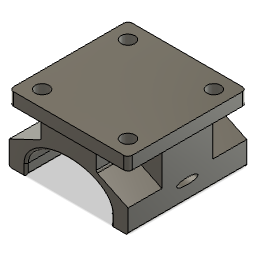
IMU_Thumb_Mount_03 v2 (Autodesk Fusion 360 design; units mm, degrees)
Autodesk Fusion 360 part; units mm, degrees
sketch "Sketch1" plane through (0, 0, 0) normal (0, 1, 0) x (1, 0, 0)
  line L0 (14, 14) -> (-14, 14)
  line L1 (-14, 14) -> (-14, -14)
  line L2 (-14, -14) -> (14, -14)
  line L3 (14, -14) -> (14, 14)
  line L4 (14, 14) -> (-14, -14) construction
  line L5 (-14, 14) -> (14, -14) construction
  line L6 (13, 13) -> (-13, 13) construction
  line L7 (-13, 13) -> (-13, -13) construction
  line L8 (-13, -13) -> (13, -13) construction
  line L9 (13, -13) -> (13, 13) construction
  line L10 (13, 13) -> (-13, -13) construction
  line L11 (-13, 13) -> (13, -13) construction
  line L12 (-10.125, 14) -> (-10.125, -14) construction
  line L13 (10.125, -14) -> (10.125, 14) construction
  line L14 (14, 10.125) -> (-14, 10.125) construction
  line L15 (-14, -10.125) -> (14, -10.125) construction
  circle A0 centre (10.125, 10.125) radius 1.625
  circle A1 centre (-10.125, 10.125) radius 1.625
  circle A2 centre (-10.125, -10.125) radius 1.625
  circle A3 centre (10.125, -10.125) radius 1.625
  dimension "d1" = 28
  dimension "d2" = 28
  dimension "d3" = 26
  dimension "d4" = 26
  dimension "d5" = 3.875
  dimension "d6" = 3.875
  dimension "d7" = 3.875
  dimension "d8" = 3.875
  dimension "d9" = 3.25
  dimension "d10" = 3.25
  dimension "d11" = 3.25
  dimension "d12" = 3.25
  constraint horizontal L0
  constraint perpendicular L0 L1
  constraint parallel L0 L2
  constraint parallel L1 L3
  constraint coincident L4 origin
  constraint coincident L5 origin
  constraint horizontal L6
  constraint perpendicular L6 L7
  constraint parallel L6 L8
  constraint parallel L7 L9
  constraint coincident L10 origin
  constraint coincident L11 origin
  constraint coincident L0 L12.start
  constraint coincident L2 L12.end
  constraint perpendicular L2 L12
  constraint coincident L2 L13.start
  constraint coincident L0 L13.end
  constraint perpendicular L0 L13
  constraint coincident L3 L14.start
  constraint perpendicular L3 L14
  constraint coincident L1 L14.end
  constraint coincident L1 L15.start
  constraint perpendicular L1 L15
  constraint coincident L3 L15.end
  constraint coincident L14 A0.centre
  constraint coincident L4 A0.centre
  constraint coincident L11 A1.centre
  constraint coincident L14 A1.centre
  constraint coincident L15 A2.centre
  constraint coincident L4 A2.centre
  constraint coincident L13 A3.centre
  constraint coincident L11 A3.centre
  measures "d1" distance of L1.end L2.end
  measures "d2" distance of L0.end L1.end
  measures "d3" distance of L7.end L8.end
  measures "d4" distance of L6.end L7.end
  measures "d5" distance of L3 L13
  measures "d6" distance of L1 L12
  measures "d7" distance of L2 L15
  measures "d8" distance of L0 L14
  measures "d9" diameter of A0
  measures "d10" diameter of A1
  measures "d11" diameter of A2
  measures "d12" diameter of A3
extrude "Extrude1" add sketch "Sketch1" along normal blind 3 makes body 1
sketch "Sketch2" plane through (0, 0, 0) normal (0, 0, 1) x (1, 0, 0)
  line L0 (0, 0) -> (0, -13) construction
  line L1 (0, 0) -> (0, -4.3333) construction
  line L2 (0, -13) -> (8.6667, -13)
  line L3 (0, -13) -> (-8.6667, -13)
  line L4 (-14, 0) -> (14, 0)
  line L5 (-8.5, 0) -> (-11.75, 0)
  line L6 (11.75, 0) -> (8.5, 0)
  line L7 (11.75, 0) -> (8.5, 0)
  line L8 (-8.5, 0) -> (-11.75, 0)
  line L9 (8.5, 0) -> (11.75, 0) construction
  line L10 (-8.5, 0) -> (-11.75, 0) construction
  line L11 (-8.5, 0) -> (-6.5, 0) construction
  line L12 (-11.75, 0) -> (-13.75, 0) construction
  line L13 (8.5, 0) -> (6.5, 0) construction
  line L14 (11.75, 0) -> (13.75, 0) construction
  line L15 (-6.5, 0) -> (-6.5, -7.1713)
  line L16 (6.5, 0) -> (6.5, -7.2675)
  line L17 (-6.5, -7.1713) -> (-13.755, -7.1713)
  line L18 (6.5, -7.2675) -> (13.8418, -7.2675)
  line L19 (0, -4.3333) -> (0, -10.3333) construction
  ellipse E0 centre (0, -10.3333) end of major axis (0, -4.3333) minor radius 10
  line L20 (0, -16.3333) -> (0, -4.3333) construction
  line L21 (10, -10.3333) -> (-10, -10.3333) construction
  line L22 (-10, -10.3333) -> (-14.8306, -10.3333) construction
  line L23 (10, -10.3333) -> (15, -10.3333) construction
  line L24 (14, 0) -> (14, -10.3333)
  line L25 (-14, 0) -> (-14, -10.3333)
  line L26 (-14, -10.3333) -> (-10, -10.3333)
  line L27 (14, -10.3333) -> (10, -10.3333)
  line L28 (-14, -10.3333) -> (-9.7808, -11.5827)
  line L29 (14, -10.3333) -> (9.781, -11.5822)
  line L30 (-13.755, -7.1713) -> (-14, -7.1713)
  line L31 (13.8418, -7.2675) -> (14, -7.2675)
  line L32 (-14, -7.1713) -> (-6.5, -3.5856)
  line L33 (14, -7.2675) -> (6.5, -3.6338)
  dimension "d15" = 13
  dimension "d16" = 4.3333
  dimension "d17" = 2
  dimension "d18" = 2
  dimension "d19" = 2
  dimension "d20" = 2
  dimension "d68" = 6
  dimension "d69" = 20
  dimension "d74" = 4.4
  constraint vertical L0
  constraint coincident L0.start L1.start
  constraint parallel L0 L1
  constraint perpendicular L0 L2
  constraint perpendicular L0 L3
  constraint horizontal L4
  constraint coincident L6.end L7.end
  constraint coincident L6.start L7.start
  constraint coincident L5.start L8.start
  constraint coincident L5.end L8.end
  constraint parallel L4 L11
  constraint parallel L4 L12
  constraint parallel L4 L13
  constraint parallel L4 L14
  constraint perpendicular L11 L15
  constraint perpendicular L13 L16
  constraint perpendicular L15 L17
  constraint perpendicular L16 L18
  constraint perpendicular L4 L19
  constraint coincident E0 L20.start
  constraint coincident E0 L1.end
  constraint coincident E0 L21.start
  constraint coincident E0 L21.end
  constraint coincident L19.end E0.centre
  constraint coincident L1.end L19.start
  constraint coincident L21.end L22.start
  constraint parallel L21 L22
  constraint coincident L21.start L23.start
  constraint parallel L21 L23
  constraint coincident L23 L24.end
  constraint perpendicular L23 L24
  constraint coincident L22 L25.end
  constraint perpendicular L22 L25
  constraint coincident E0 L28.end
  constraint coincident E0 L29.end
  constraint coincident L25 L30.end
  constraint perpendicular L25 L30
  constraint coincident L24 L31.end
  constraint perpendicular L24 L31
  constraint midpoint L15 L32.end
  constraint midpoint L16 L33.end
  measures "d15" distance of L0.start L0.end
  measures "d16" distance of L0.start L1.end
  measures "d17" distance of L5.start L11.end
  measures "d18" distance of L5.end L12.end
  measures "d19" distance of L6.end L13.end
  measures "d20" distance of L6.start L14.end
  measures "d68" distance of L1.end L19.end
  measures "d74" distance of L24.end L29.end
extrude "Extrude11" add sketch "Sketch2" along normal mid plane 12 separate body contours L4 L5 L8 L15 L25 L32 | L15 L17 E0 L30 L32 | L4 L15 L16 E0 | L4 L6 L7 L16 L24 L33 | L16 L18 E0 L31 L33 | L18 E0 L24 L27 L31 makes body 2
extrude "Extrude12" add sketch "Sketch2" along normal mid plane 28 separate body contours L17 E0 L25 L26 L30 | L15 L17 E0 L30 L32 | L4 L15 L16 E0 | L16 L18 E0 L31 L33 | L18 E0 L24 L27 L31 makes body 3
sketch "Sketch4" plane through (-14, 0, 0) normal (-1, 0, 0) x (0, 0, 1)
  line L0 (-14, -10.3333) -> (14, -10.3333)
  line L1 (14, -10.3333) -> (14, -7.1713)
  line L2 (-14, -7.1713) -> (-14, -10.3333)
  line L3 (0, 0) -> (0, -10.3333)
  line L4 (0, -7.1713) -> (0, -10.3333) construction
  ellipse E0 centre (0, -8.7523) end of major axis (0, -9.5023) minor radius 2.5
  line L5 (0, -8.0023) -> (0, -9.5023) construction
  line L6 (-2.5, -8.7523) -> (2.5, -8.7523) construction
  line L7 (-14, -10.3333) -> (14, -10.3333)
  line L8 (14, -10.3333) -> (14, -12.8333)
  line L9 (14, -12.8333) -> (-14, -12.8333)
  line L10 (-14, -12.8333) -> (-14, -10.3333)
  line L11 (14, -7.1713) -> (-14, -7.1713)
  dimension "d75" = 1.5
  dimension "d76" = 5
  dimension "d83" = 2.5
  constraint coincident L3.end L4.end
  constraint coincident E0 L5.start
  constraint coincident E0 L5.end
  constraint coincident E0 L6.start
  constraint coincident E0 L6.end
  constraint midpoint L4 E0.centre
  constraint horizontal L7
  constraint vertical L8
  constraint horizontal L9
  constraint vertical L10
  constraint coincident L0.start L2.end
  measures "d75" distance of E0
  measures "d83" distance of L0.start L9.end
extrude "Extrude13" cut sketch "Sketch4" against normal blind 28 contours L3 E0 | L3 E0 bodies 2 3
fillet "Fillet15" radius 1 4 edges at (14, 1.5, -14) (-14, 1.5, -14) (-14, 1.5, 14) (14, 1.5, 14) on bodies 1
extrude "Extrude14" add sketch "Sketch4" against normal blind 4 contours L0 L7 L8 L9 L10 bodies 3
sketch "Sketch5" plane through (14, 0, 0) normal (1, 0, 0) x (0, 0, -1)
  line L0 (-14, -10.3333) -> (14, -10.3333)
  ellipse E0 centre (0, -8.7523) end of major axis (-2.5, -8.7523) minor radius 0.75
  line L1 (-14, -12.8333) -> (14, -12.8333)
  line L2 (14, -12.8333) -> (14, -10.3333)
  line L3 (-14, -10.3333) -> (-14, -12.8333)
  line L4 (-14, -10.3333) -> (14, -10.3333)
  line L5 (14, -10.3333) -> (14, -12.8333)
  line L6 (14, -12.8333) -> (-14, -12.8333)
  line L7 (-14, -12.8333) -> (-14, -10.3333)
  line L8 (-14, -7.2675) -> (-14, -10.3333)
  line L9 (14, -10.3333) -> (14, -7.2675)
  line L10 (14, -10.3333) -> (-14, -10.3333)
  line L11 (14, -7.2675) -> (-14, -7.2675)
  constraint horizontal L4
  constraint vertical L5
  constraint horizontal L6
  constraint vertical L7
  constraint coincident L1.end L2.start
  constraint coincident L0.start L3.start
extrude "Extrude15" add sketch "Sketch5" against normal blind 4 contours L0 L1 L2 L3 L4 L5 L6 L7 L10 bodies 2 3
fillet "Fillet16" radius 0.5 10 edges at (10, -11.5833, -14) (0, -4.3333, -14) (-10, -11.5833, -14) (-10, -11.5833, 14) (0, -4.3333, 14) (10, -11.5833, 14) (-14, -12.8333, 0) (-10, -12.8333, 0) (10, -12.8333, 0) (14, -12.8333, 0) on bodies 2
fillet "Fillet17" radius 0.5 4 edges at (6.5, -3.6338, 10) (6.5, -3.6338, -10) (-6.5, -3.5856, -10) (-6.5, -3.5856, 10) on bodies 2
equation "d16 = ( 13 / 3 ) * 1 mm"
